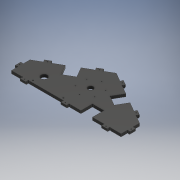
# Autodesk Inventor part: BA07
Saved by Autodesk Inventor 2017 (Build 210142000, 142)
## iProperties
Created: 2019-05-24
Part Number: BA07
Material: Wood (Cherry)
Document SubType Name: Modeling
Designer: Dell
Density: 0.63 g/cm^3
Appearance: Smooth - Black
Mass: 565.211 g
Surface Area: 1690.7 cm^2
Volume: 897.161 cm^3
Author: Dell
Autodesk Inventor part; units mm, degrees
ref_plane "YZ Plane" through (0, 0, 0) normal (1, 0, 0) x (0, 1, 0)
ref_plane "XZ Plane" through (0, 0, 0) normal (0, 1, 0) x (-1, 0, 0)
ref_plane "XY Plane" through (0, 0, 0) normal (0, 0, 1) x (1, 0, 0)
sketch "Sketch1" plane through (0, 0, 0) normal (0, 0, 1) x (1, 0, 0)
  line L0 (0, 0) -> (0, 101.6)
  line L1 (0, 0) -> (525.78, 0)
  line L2 (525.78, 0) -> (525.78, 101.6)
  line L3 (525.78, 101.6) -> (262.89, 253.3796)
  line L4 (262.89, 253.3796) -> (0, 101.6)
  line L5 (10.795, 95.3675) -> (10.795, 10.795)
  line L6 (10.795, 10.795) -> (514.985, 10.795)
  line L7 (514.985, 10.795) -> (514.985, 95.3675)
  line L8 (514.985, 95.3675) -> (262.89, 240.9146)
  line L9 (262.89, 240.9146) -> (10.795, 95.3675)
  point P0 (262.89, 0)
  dimension "d0" = 101.6
  dimension "d1" = 525.78
  dimension "d2" = 120
  dimension "d3" = 10.795
  constraints: 20 end point, 2 perpendicular, 1 horizontal, 1 horizontal alignment, 1 midpoint, 1 vertical, 1 vertical alignment, 4 other
  measures "d0" distance of L0.start L0.end
  measures "d1" distance of L0.start L1.end
  measures "d2" angle of L0 L4
  measures "d3" distance between parallel lines of L4 L9
extrude "Extrusion1" add sketch "Sketch1" along normal blind 9.525 contours L9 L8 L7 L6 L5
sketch "Sketch2" plane through (0, 0, 9.525) normal (0, 0, 1) x (1, 0, 0)
  line L0 (10.795, 95.3675) -> (10.795, 10.795)
  line L1 (10.795, 65.5129) -> (1.27, 65.5129)
  line L2 (1.27, 65.5129) -> (1.27, 40.1129)
  line L3 (1.27, 40.1129) -> (10.795, 40.1129)
  line L4 (10.795, 40.1129) -> (10.795, 65.5129)
  line L5 (514.985, 65.5129) -> (524.51, 65.5129)
  line L6 (524.51, 65.5129) -> (524.51, 40.1129)
  line L7 (524.51, 40.1129) -> (514.985, 40.1129)
  line L8 (514.985, 40.1129) -> (514.985, 65.5129)
  line L9 (514.985, 10.795) -> (514.985, 95.3675) projected
  line L10 (10.795, 10.795) -> (514.985, 10.795) projected
  line L11 (62.69, 10.795) -> (88.09, 10.795)
  line L12 (88.09, 10.795) -> (88.09, 1.27)
  line L13 (88.09, 1.27) -> (62.69, 1.27)
  line L14 (62.69, 1.27) -> (62.69, 10.795)
  line L15 (250.19, 10.795) -> (275.59, 10.795)
  line L16 (275.59, 10.795) -> (275.59, 1.27)
  line L17 (275.59, 1.27) -> (250.19, 1.27)
  line L18 (250.19, 1.27) -> (250.19, 10.795)
  line L19 (437.69, 10.795) -> (463.09, 10.795)
  line L20 (463.09, 10.795) -> (463.09, 1.27)
  line L21 (463.09, 1.27) -> (437.69, 1.27)
  line L22 (437.69, 1.27) -> (437.69, 10.795)
  line L23 (75.39, 1.27) -> (450.39, 1.27) construction
  line L24 (50.0668, 118.0411) -> (45.3043, 126.29)
  line L25 (45.3043, 126.29) -> (67.3013, 138.99)
  line L26 (67.3013, 138.99) -> (72.0638, 130.7411)
  line L27 (72.0638, 130.7411) -> (50.0668, 118.0411)
  line L28 (201.6212, 205.5411) -> (196.8587, 213.79)
  line L29 (196.8587, 213.79) -> (218.8557, 226.49)
  line L30 (218.8557, 226.49) -> (223.6182, 218.2411)
  line L31 (223.6182, 218.2411) -> (201.6212, 205.5411)
  line L32 (262.89, 240.9146) -> (10.795, 95.3675) projected
  line L33 (56.3028, 132.64) -> (207.8572, 220.14) construction
  line L34 (132.08, 176.39) -> (136.8425, 168.1411)
  line L35 (514.985, 95.3675) -> (262.89, 240.9146) projected
  line L36 (262.89, 240.9146) -> (262.89, 274.3369)
  line L37 (475.7132, 118.0411) -> (480.4757, 126.29)
  line L38 (480.4757, 126.29) -> (458.4787, 138.99)
  line L39 (458.4787, 138.99) -> (453.7162, 130.7411)
  line L40 (453.7162, 130.7411) -> (475.7132, 118.0411)
  line L41 (324.1588, 205.5411) -> (328.9213, 213.79)
  line L42 (328.9213, 213.79) -> (306.9243, 226.49)
  line L43 (306.9243, 226.49) -> (302.1618, 218.2411)
  line L44 (302.1618, 218.2411) -> (324.1588, 205.5411)
  line L45 (469.4772, 132.64) -> (317.9228, 220.14) construction
  line L46 (393.7, 176.39) -> (388.9375, 168.1411)
  circle A0 centre (519.7475, 52.8129) radius 2.25
  circle A1 centre (467.096, 128.5155) radius 2.25
  circle A2 centre (450.39, 6.0325) radius 2.25
  circle A3 centre (262.89, 6.0325) radius 2.25
  circle A4 centre (75.39, 6.0325) radius 2.25
  circle A5 centre (6.0325, 52.8129) radius 2.25
  circle A6 centre (58.684, 128.5155) radius 2.25
  circle A7 centre (210.2385, 216.0155) radius 2.25
  circle A8 centre (315.5415, 216.0155) radius 2.25
  line L47 (58.684, 128.5155) -> (56.3028, 132.64) construction
  line L48 (58.684, 128.5155) -> (69.6825, 134.8655) construction
  line L49 (199.24, 209.6655) -> (210.2385, 216.0155) construction
  line L50 (210.2385, 216.0155) -> (207.8572, 220.14) construction
  line L51 (326.54, 209.6655) -> (315.5415, 216.0155) construction
  line L52 (315.5415, 216.0155) -> (317.9228, 220.14) construction
  line L53 (456.0975, 134.8655) -> (467.096, 128.5155) construction
  line L54 (467.096, 128.5155) -> (469.4772, 132.64) construction
  line L55 (9.525, 96.1007) -> (9.525, 9.525) construction
  line L56 (9.525, 9.525) -> (516.255, 9.525) construction
  line L57 (516.255, 9.525) -> (516.255, 96.1007) construction
  line L58 (516.255, 96.1007) -> (262.89, 242.3811) construction
  line L59 (262.89, 242.3811) -> (9.525, 96.1007) construction
  point P0 (0, 0)
  point P1 (262.89, 10.795)
  point P2 (262.89, 1.27)
  point P3 (262.89, 10.795)
  point P4 (88.09, 6.0325)
  point P5 (250.19, 6.0325)
  point P6 (437.69, 6.0325)
  point P7 (6.0325, 65.5129)
  point P8 (75.39, 10.795)
  point P9 (262.89, 10.795)
  point P10 (450.39, 10.795)
  point P11 (519.7475, 65.5129)
  point P12 (9.525, 52.8129)
  point P13 (1.27, 52.8129)
  point P14 (516.255, 52.8129)
  point P15 (524.51, 52.8129)
  dimension "d6" = 9.525
  dimension "d7" = 25.4
  dimension "d8" = 9.525
  dimension "d9" = 25.4
  dimension "d10" = 25.4
  dimension "d11" = 9.525
  dimension "d12" = 25.4
  dimension "d13" = 9.525
  dimension "d14" = 25.4
  dimension "d15" = 9.525
  dimension "d16" = 375
  dimension "d17" = 25.4
  dimension "d18" = 9.525
  dimension "d19" = 9.525
  dimension "d20" = 25.4
  dimension "d21" = 175
  dimension "d28" = 4.5
  dimension "d29" = 4.5
  dimension "d30" = 4.5
  dimension "d31" = 4.5
  dimension "d32" = 4.5
  dimension "d33" = 4.5
  dimension "d34" = 4.5
  dimension "d35" = 4.5
  dimension "d36" = 4.5
  dimension "d112" = 1.27
  constraints: 112 end point, 23 midpoint, 16 perpendicular, 14 parallel, 12 symmetric about line, 9 centre point, 7 horizontal alignment, 7 point on line, 6 vertical alignment, 5 horizontal, 1 vertical, 12 other
  measures "d6" distance of L3.end L2.end
  measures "d7" distance of L2.end L1.end
  measures "d8" distance of L6.end L7.end
  measures "d9" distance of L5.end L6.end
  measures "d10" distance of L12.end L13.end
  measures "d11" distance of L11.end L12.end
  measures "d12" distance of L16.end L17.end
  measures "d13" distance of L15.end L16.end
  measures "d14" distance of L20.end L21.end
  measures "d15" distance of L19.end L20.end
  measures "d16" distance of L23.start L23.end
  measures "d17" distance of L28.end L29.end
  measures "d18" distance of L29.end L30.end
  measures "d19" distance of L24.start L24.end
  measures "d20" distance of L24.end L25.end
  measures "d21" distance of L33.start L33.end
  measures "d28" diameter of A0
  measures "d29" diameter of A1
  measures "d30" diameter of A2
  measures "d31" diameter of A3
  measures "d32" diameter of A4
  measures "d33" diameter of A5
  measures "d34" diameter of A6
  measures "d35" diameter of A7
  measures "d36" diameter of A8
  measures "d112" distance between parallel lines of L32 L59
extrude "Extrusion2" add sketch "Sketch2" against normal blind 12.7
sketch "Sketch3" plane through (0, 0, 9.525) normal (0, 0, 1) x (1, 0, 0)
  circle A0 centre (262.89, 122.6496) radius 60
  line L0 (250.19, 1.27) -> (275.59, 1.27) projected
  point P0 (0, 0)
  point P1 (262.89, 1.27)
  dimension "d24" = 120
  dimension "d25" = 121.3796
  constraints: 1 centre point, 1 midpoint, 1 vertical alignment
  measures "d24" diameter of A0
  measures "d25" distance from line of L0 A0.centre
extrude "Extrusion3" cut sketch "Sketch3" against normal through all
sketch "Sketch5" plane through (0, 0, 9.525) normal (0, 0, 1) x (1, 0, 0)
  line L0 (437.69, 10.795) -> (275.59, 10.795) projected
  line L1 (329.97, 10.795) -> (383.31, 10.795)
  line L2 (383.31, 10.795) -> (383.31, 64.135)
  line L3 (383.31, 64.135) -> (329.97, 64.135)
  line L4 (329.97, 64.135) -> (329.97, 10.795)
  point P0 (0, 0)
  point P1 (356.64, 10.795)
  dimension "d37" = 53.34
  dimension "d38" = 53.34
  constraints: 8 end point, 2 midpoint, 2 parallel, 1 horizontal, 1 perpendicular, 1 point on line
  measures "d37" distance of L3.end L2.end
  measures "d38" distance of L2.end L1.end
extrude "Extrusion4" cut sketch "Sketch5" against normal through all
sketch "Sketch6" plane through (0, 0, 9.525) normal (0, 0, 1) x (1, 0, 0)
  line L0 (159.9394, 181.4761) -> (186.6094, 135.2823)
  line L1 (186.6094, 135.2823) -> (140.4156, 108.6123)
  line L2 (140.4156, 108.6123) -> (113.7456, 154.8061)
  line L3 (113.7456, 154.8061) -> (159.9394, 181.4761)
  line L4 (453.7162, 130.7411) -> (324.1588, 205.5411) projected
  line L5 (412.0344, 154.8061) -> (385.3644, 108.6123)
  line L6 (385.3644, 108.6123) -> (339.1706, 135.2823)
  line L7 (339.1706, 135.2823) -> (365.8406, 181.4761)
  line L8 (365.8406, 181.4761) -> (412.0344, 154.8061)
  line L9 (201.6212, 205.5411) -> (72.0638, 130.7411) projected
  point P0 (0, 0)
  point P1 (136.8425, 168.1411)
  point P2 (388.9375, 168.1411)
  dimension "d41" = 53.34
  dimension "d42" = 53.34
  dimension "d43" = 53.34
  dimension "d44" = 53.34
  constraints: 16 end point, 4 midpoint, 4 parallel, 4 point on line, 2 perpendicular
  measures "d41" distance of L5.end L6.end
  measures "d42" distance of L5.start L5.end
  measures "d43" distance of L0.end L1.end
  measures "d44" distance of L0.start L0.end
extrude "Extrusion5" cut sketch "Sketch6" against normal through all
sketch "Sketch7" plane through (0, 0, 9.525) normal (0, 0, 1) x (1, 0, 0)
  circle A0 centre (262.89, 173.6496) radius 2
  circle A1 centre (262.89, 122.6496) radius 60 projected
  circle A2 centre (262.89, 122.6496) radius 12.5
  circle A3 centre (262.89, 122.6496) radius 12.5
  circle A4 centre (218.7227, 148.1496) radius 2
  circle A5 centre (262.89, 122.6496) radius 12.5
  circle A6 centre (218.7227, 97.1496) radius 2
  circle A7 centre (262.89, 122.6496) radius 12.5
  circle A8 centre (262.89, 71.6496) radius 2
  circle A9 centre (262.89, 122.6496) radius 12.5
  circle A10 centre (307.0573, 97.1496) radius 2
  circle A11 centre (262.89, 122.6496) radius 12.5
  circle A12 centre (307.0573, 148.1496) radius 2
  point P0 (0, 0)
  dimension "d47" = 4
  dimension "d48" = 51
  dimension "d49" = 25
  dimension "d52" = 360
  constraints: 12 centre point, 1 coincident, 1 vertical alignment, 25 other
  measures "d47" diameter of A0
  measures "d48" distance of A1.centre A0.centre
  measures "d49" diameter of A2
extrude "Extrusion6" add sketch "Sketch7" against normal blind 12.7
sketch "Sketch8" plane through (0, 0, 9.525) normal (0, 0, 1) x (1, 0, 0)
  circle A0 centre (110.795, 60.795) radius 15
  line L0 (88.09, 10.795) -> (250.19, 10.795) projected
  line L1 (10.795, 40.1129) -> (10.795, 10.795) projected
  point P0 (0, 0)
  dimension "d56" = 30
  dimension "d57" = 50
  dimension "d58" = 100
  constraints: 1 centre point
  measures "d56" diameter of A0
  measures "d57" distance from line of L0 A0.centre
  measures "d58" distance from line of L1 A0.centre
extrude "Extrusion7" cut sketch "Sketch8" against normal through all
sketch "Sketch9" plane through (0, 0, 9.525) normal (0, 0, 1) x (1, 0, 0)
  line L0 (250.19, 10.795) -> (88.09, 10.795) construction
  line L1 (88.09, 10.795) -> (110.19, 10.795) construction
  line L2 (110.19, 10.795) -> (110.19, 30.795) construction
  line L3 (110.19, 30.795) -> (88.09, 30.795) construction
  line L4 (88.09, 30.795) -> (88.09, 10.795) construction
  line L5 (250.19, 10.795) -> (228.09, 10.795) construction
  line L6 (228.09, 10.795) -> (228.09, 30.795) construction
  line L7 (228.09, 30.795) -> (250.19, 30.795) construction
  line L8 (250.19, 30.795) -> (250.19, 10.795) construction
  circle A0 centre (99.14, 20.795) radius 3
  circle A1 centre (239.14, 20.795) radius 3
  point P0 (0, 0)
  point P1 (99.14, 30.795)
  point P2 (239.14, 30.795)
  point P3 (110.19, 20.795)
  point P4 (228.09, 20.795)
  dimension "d62" = 20
  dimension "d64" = 20
  dimension "d65" = 6
  dimension "d66" = 6
  dimension "d69" = 11.05
  dimension "d70" = 11.05
  constraints: 16 end point, 4 midpoint, 4 parallel, 2 centre point, 2 horizontal, 2 horizontal alignment, 2 perpendicular, 2 vertical alignment
  measures "d62" distance of L2.end L1.end
  measures "d64" distance of L5.end L6.end
  measures "d65" diameter of A0
  measures "d66" diameter of A1
  measures "d69" horizontal distance of L0.end A0.centre
  measures "d70" horizontal distance of L0.start A1.centre
extrude "Extrusion8" cut sketch "Sketch9" against normal through all
sketch "Sketch10" plane through (0, 0, 9.525) normal (0, 0, 1) x (1, 0, 0)
  circle A0 centre (8.5499, 67.7579) radius 3.175
  circle A1 centre (8.5499, 37.8678) radius 3.175
  circle A2 centre (60.4449, 8.5499) radius 3.175
  circle A3 centre (90.3351, 8.5499) radius 3.175
  circle A4 centre (247.9449, 8.5499) radius 3.175
  circle A5 centre (277.8351, 8.5499) radius 3.175
  circle A6 centre (435.4449, 8.5499) radius 3.175
  circle A7 centre (465.3351, 8.5499) radius 3.175
  circle A8 centre (517.2301, 37.8678) radius 3.175
  circle A9 centre (517.2301, 67.7579) radius 3.175
  circle A10 centre (478.7801, 118.8628) radius 3.175
  circle A11 centre (452.8944, 133.8079) radius 3.175
  circle A12 centre (327.2256, 206.3628) radius 3.175
  circle A13 centre (301.34, 221.3079) radius 3.175
  circle A14 centre (224.44, 221.3079) radius 3.175
  circle A15 centre (198.5544, 206.3628) radius 3.175
  circle A16 centre (72.8856, 133.8079) radius 3.175
  circle A17 centre (46.9999, 118.8628) radius 3.175
  line L0 (60.4449, 8.5499) -> (62.69, 10.795)
  line L1 (10.795, 10.795) -> (62.69, 10.795)
  line L2 (10.795, 65.5129) -> (8.5499, 67.7579)
  line L3 (10.795, 95.3675) -> (10.795, 65.5129)
  line L4 (514.985, 65.5129) -> (517.2301, 67.7579)
  line L5 (514.985, 65.5129) -> (524.51, 65.5129)
  line L6 (475.7132, 118.0411) -> (478.7801, 118.8628)
  line L7 (478.7801, 118.8628) -> (301.34, 221.3079)
  line L8 (514.985, 95.3675) -> (475.7132, 118.0411)
  line L9 (365.8406, 181.4761) -> (324.1588, 205.5411)
  line L10 (45.3043, 126.29) -> (50.0668, 118.0411)
  line L11 (50.0668, 118.0411) -> (46.9999, 118.8628)
  line L12 (46.9999, 118.8628) -> (224.44, 221.3079)
  line L13 (201.6212, 205.5411) -> (159.9394, 181.4761)
  line L14 (1.27, 40.1129) -> (10.795, 40.1129) projected
  point P0 (0, 0)
  point P1 (0, 0)
  point P2 (88.09, 10.795)
  point P3 (250.19, 10.795)
  point P4 (275.59, 10.795)
  point P5 (437.69, 10.795)
  point P6 (463.09, 10.795)
  point P7 (72.0638, 130.7411)
  point P8 (223.6182, 218.2411)
  point P9 (302.1618, 218.2411)
  point P10 (453.7162, 130.7411)
  point P11 (514.985, 40.1129)
  point P12 (88.09, 10.795)
  point P13 (250.19, 10.795)
  point P14 (275.59, 10.795)
  point P15 (72.0638, 130.7411)
  point P16 (223.6182, 218.2411)
  point P17 (302.1618, 218.2411)
  point P18 (453.7162, 130.7411)
  point P19 (514.985, 40.1129)
  point P20 (463.09, 10.795)
  point P21 (437.69, 10.795)
  dimension "d71" = 6.35
  dimension "d72" = 6.35
  dimension "d73" = 6.35
  dimension "d74" = 6.35
  dimension "d75" = 6.35
  dimension "d76" = 6.35
  dimension "d77" = 6.35
  dimension "d78" = 6.35
  dimension "d79" = 6.35
  dimension "d80" = 6.35
  dimension "d81" = 6.35
  dimension "d82" = 6.35
  dimension "d83" = 6.35
  dimension "d84" = 6.35
  dimension "d85" = 6.35
  dimension "d86" = 6.35
  dimension "d87" = 6.35
  dimension "d88" = 6.35
  dimension "d89" = 45
  dimension "d90" = 45
  dimension "d91" = 45
  dimension "d92" = 45
  dimension "d93" = 45
  constraints: 28 end point, 24 coincident, 5 horizontal alignment, 4 point on line, 2 parallel, 2 vertical alignment, 1 perpendicular, 54 other
  measures "d89" angle of L1 L0
  measures "d90" angle of L3 L2
  measures "d91" angle of L5 L4
  measures "d92" angle of L6 L8
  measures "d93" angle of L10 L11
extrude "Extrusion9" cut sketch "Sketch10" against normal through all
sketch "Sketch11" plane through (0, 0, 9.525) normal (0, 0, 1) x (1, 0, 0)
  circle A0 centre (141.2374, 111.6791) radius 3.175
  circle A1 centre (183.5426, 136.104) radius 3.175
  circle A2 centre (342.2374, 136.104) radius 3.175
  circle A3 centre (384.5426, 111.6791) radius 3.175
  circle A4 centre (332.2151, 61.8899) radius 3.175
  circle A5 centre (381.0649, 61.8899) radius 3.175
  line L0 (140.4156, 108.6123) -> (113.7456, 154.8061)
  line L1 (140.4156, 108.6123) -> (141.2374, 111.6791)
  line L2 (141.2374, 111.6791) -> (183.5426, 136.104)
  line L3 (339.1706, 135.2823) -> (385.3644, 108.6123)
  line L4 (339.1706, 135.2823) -> (342.2374, 136.104)
  line L5 (342.2374, 136.104) -> (384.5426, 111.6791)
  line L6 (383.31, 64.135) -> (329.97, 64.135)
  line L7 (329.97, 64.135) -> (332.2151, 61.8899)
  line L8 (332.2151, 61.8899) -> (381.0649, 61.8899)
  line L9 (186.6094, 135.2823) -> (140.4156, 108.6123)
  point P0 (0, 0)
  point P1 (0, 0)
  dimension "d96" = 6.35
  dimension "d100" = 6.35
  dimension "d101" = 6.35
  dimension "d102" = 6.35
  dimension "d103" = 6.35
  dimension "d104" = 6.35
  dimension "d97" = 45
  dimension "d98" = 45
  dimension "d99" = 45
  constraints: 20 end point, 7 coincident, 2 parallel, 1 horizontal, 18 other
  measures "d97" angle of L9 L1
  measures "d98" angle of L3 L4
  measures "d99" angle of L6 L7
extrude "Extrusion10" cut sketch "Sketch11" against normal through all contours A0 L9 L1 L2 | L2 L1 L0 A0 | A0 L9 | L0 A0 | A1 L9 | L9 A1 | A2 L5 L4 | L3 A2 | L4 L5 A2 L3 | A3 L3 | L3 A3 | L7 L8 A4 | A4 L6 | L6 A4 L8 L7 | A5 L6 | A5 L6
sketch "Sketch12" plane through (0, 0, 9.525) normal (0, 0, 1) x (1, 0, 0)
  line L0 (45.3043, 126.29) -> (67.3013, 138.99) projected
  line L1 (45.3043, 126.29) -> (44.0343, 128.4897)
  line L2 (44.0343, 128.4897) -> (66.0313, 141.1897)
  line L3 (66.0313, 141.1897) -> (67.3013, 138.99)
  line L4 (67.3013, 138.99) -> (45.3043, 126.29)
  line L5 (196.8587, 213.79) -> (218.8557, 226.49) projected
  line L6 (218.8557, 226.49) -> (217.5857, 228.6897)
  line L7 (217.5857, 228.6897) -> (195.5887, 215.9897)
  line L8 (195.5887, 215.9897) -> (196.8587, 213.79)
  line L9 (196.8587, 213.79) -> (218.8557, 226.49)
  line L10 (1.27, 40.1129) -> (1.27, 65.5129) projected
  line L11 (1.27, 40.1129) -> (-1.27, 40.1129)
  line L12 (-1.27, 40.1129) -> (-1.27, 65.5129)
  line L13 (-1.27, 65.5129) -> (1.27, 65.5129)
  line L14 (1.27, 65.5129) -> (1.27, 40.1129)
  line L15 (62.69, 1.27) -> (62.69, 6.3049) projected
  line L16 (62.69, 1.27) -> (88.09, 1.27)
  line L17 (88.09, 1.27) -> (88.09, -1.27)
  line L18 (88.09, -1.27) -> (62.69, -1.27)
  line L19 (62.69, -1.27) -> (62.69, 1.27)
  line L20 (250.19, 1.27) -> (275.59, 1.27) projected
  line L21 (275.59, 1.27) -> (250.19, 1.27)
  line L22 (250.19, 1.27) -> (250.19, -1.27)
  line L23 (250.19, -1.27) -> (275.59, -1.27)
  line L24 (275.59, -1.27) -> (275.59, 1.27)
  line L25 (298.2732, 220.4861) -> (262.89, 240.9146) projected
  line L26 (262.89, 240.9146) -> (262.89, 275.9262)
  line L27 (480.4757, 126.29) -> (458.4787, 138.99)
  line L28 (480.4757, 126.29) -> (481.7457, 128.4897)
  line L29 (481.7457, 128.4897) -> (459.7487, 141.1897)
  line L30 (459.7487, 141.1897) -> (458.4787, 138.99)
  line L31 (458.4787, 138.99) -> (480.4757, 126.29)
  line L32 (328.9213, 213.79) -> (306.9243, 226.49)
  line L33 (306.9243, 226.49) -> (308.1943, 228.6897)
  line L34 (308.1943, 228.6897) -> (330.1913, 215.9897)
  line L35 (330.1913, 215.9897) -> (328.9213, 213.79)
  line L36 (328.9213, 213.79) -> (306.9243, 226.49)
  line L37 (524.51, 40.1129) -> (524.51, 65.5129)
  line L38 (524.51, 40.1129) -> (527.05, 40.1129)
  line L39 (527.05, 40.1129) -> (527.05, 65.5129)
  line L40 (527.05, 65.5129) -> (524.51, 65.5129)
  line L41 (524.51, 65.5129) -> (524.51, 40.1129)
  line L42 (463.09, 1.27) -> (463.09, 6.3049)
  line L43 (463.09, 1.27) -> (437.69, 1.27)
  line L44 (437.69, 1.27) -> (437.69, -1.27)
  line L45 (437.69, -1.27) -> (463.09, -1.27)
  line L46 (463.09, -1.27) -> (463.09, 1.27)
  point P0 (0, 0)
  point P1 (525.78, 0)
  dimension "d107" = 2.54
  dimension "d108" = 2.54
  dimension "d109" = 2.54
  constraints: 82 end point, 19 symmetric about line, 10 parallel, 7 perpendicular, 3 horizontal, 2 coincident, 2 point on line, 1 horizontal alignment, 1 vertical
  measures "d107" distance of L0.start L1.end
  measures "d108" distance of L12.end L10.end
  measures "d109" distance of L18.end L15.start
extrude "Extrusion11" add sketch "Sketch12" against normal blind 9.525
equation "\"d3\" = Panel_Thickness + Fit_Tolerance"
equation "\"d4\" = Panel_Thickness"
equation "\"d6\" = d11"
equation "\"d8\" = d11"
equation "\"d9\" = d7"
equation "\"d10\" = d7"
equation "\"d11\" = Panel_Thickness"
equation "\"d12\" = d7"
equation "\"d13\" = d11"
equation "\"d14\" = d7"
equation "\"d15\" = d13"
equation "\"d17\" = d7"
equation "\"d18\" = d11"
equation "\"d19\" = d11"
equation "\"d20\" = d7"
equation "\"d112\" = Fit_Tolerance"
equation "\"d38\" = d37"
equation "\"d41\" = d43"
equation "\"d42\" = d41"
equation "\"d44\" = d43"
equation "\"d71\" = Tool_Dia"
equation "\"d72\" = d71"
equation "\"d73\" = d72"
equation "\"d74\" = d73"
equation "\"d75\" = d74"
equation "\"d76\" = d75"
equation "\"d77\" = d76"
equation "\"d78\" = d71"
equation "\"d79\" = d77"
equation "\"d80\" = d77"
equation "\"d81\" = d79"
equation "\"d82\" = d79"
equation "\"d83\" = d82"
equation "\"d84\" = d83"
equation "\"d85\" = d84"
equation "\"d86\" = d85"
equation "\"d87\" = d86"
equation "\"d88\" = d87"
equation "\"d96\" = Tool_Dia"
equation "\"d100\" = d96"
equation "\"d101\" = d100"
equation "\"d102\" = d101"
equation "\"d103\" = d102"
equation "\"d104\" = d102"
equation "\"d107\" = 2 * Fit_Tolerance"
equation "\"d108\" = 2 * Fit_Tolerance"
equation "\"d109\" = 2 * Fit_Tolerance"
equation "\"d110\" = Panel_Thickness"
equation "\"Panel_Thickness\" = 9.525"
equation "\"Fit_Tolerance\" = 1.27"
equation "\"Tool_Dia\" = 6.35"
body "Solid1"
